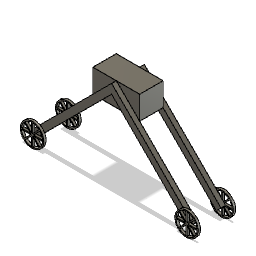
test_5 v1 (Autodesk Fusion 360 design; units mm, degrees)
Autodesk Fusion 360 part; units mm, degrees
sketch "Sketch1" plane through (0, 0, 0) normal (0, 0, 1) x (1, 0, 0)
  line L0 (0, 0) -> (200, 0)
  line L1 (200, 0) -> (200, 100)
  line L2 (200, 100) -> (0, 100)
  line L3 (0, 100) -> (0, 0)
  dimension "d1" = 200
  dimension "d2" = 100
  constraint horizontal L0
  constraint vertical L1
  constraint horizontal L2
  constraint vertical L3
  constraint coincident L0.start L3.end
  measures "d1" distance of L0.start L0.end
  measures "d2" distance of L0.start L2.end
extrude "Extrude1" add sketch "Sketch1" along normal blind 100 makes body 1
move_body "Move1" bodies 1 to x (1, 0, 0) y (0, 1, 0) z (0, 0, 1) at (0, 300, 0)
sketch "Sketch2" plane through (0, 0, 100) normal (0, 0, 1) x (1, 0, 0)
  line L0 (0, 400) -> (0, 300)
  line L1 (0, 300) -> (200, 300)
  line L2 (200, 300) -> (200, 400)
  line L3 (200, 400) -> (0, 400)
  line L4 (100, 400) -> (200, 300)
  line L5 (90, 390) -> (100, 400)
  line L6 (200, 300) -> (190, 290)
  line L7 (100, 400) -> (80, 420)
  line L8 (80, 420) -> (70, 410)
  line L9 (90, 390) -> (0, 300)
  line L10 (100, 400) -> (120, 420)
  line L11 (120, 420) -> (130, 410)
  line L12 (10, 290) -> (0, 300)
  line L13 (190, 290) -> (180, 280)
  line L14 (180, 280) -> (60, 400)
  line L15 (70, 410) -> (60, 400)
  line L16 (130, 410) -> (140, 400)
  line L17 (20, 280) -> (10, 290)
  line L18 (20, 280) -> (140, 400)
  constraint midpoint L3 L4.start
  constraint coincident L1.end L2.start
  constraint perpendicular L4 L5
  constraint perpendicular L5 L7
  constraint perpendicular L7 L8
  constraint coincident L0.end L1.start
  constraint perpendicular L7 L10
  constraint perpendicular L10 L11
  constraint perpendicular L9 L12
  constraint coincident L3 L14.end
  constraint perpendicular L13 L14
  constraint perpendicular L14 L15
  constraint coincident L3 L16.end
  constraint perpendicular L16 L18
extrude "Extrude2" add sketch "Sketch2" along normal blind 20 separate body contours L1 L9 L14 L18 | L1 L12 L17 L18 | L4 L5 L9 L14 L18 | L1 L4 L14 L18 | L1 L6 L13 L14 makes body 2
extrude "Extrude3" add 2 faces at (186.6667, 286.6667, 106.6667) (196.6667, 296.6667, 106.6667) along direction (0.707107, -0.707107, 0) blind 350 separate body on bodies 2 makes body 3
extrude "Extrude4" add 2 faces at (6.6667, 293.3333, 113.3333) (16.6667, 283.3333, 106.6667) along direction (-0.707107, -0.707107, 0) blind 350 separate body on bodies 2 makes body 4
combine "Combine1" operation add target body 4 tool bodies 3 2
sketch "Sketch3" plane through (0, 0, 120) normal (0, 0, 1) x (1, 0, 0)
  line L0 (100, 400) -> (-247.4874, 52.5126)
  line L1 (-247.4874, 52.5126) -> (-227.4874, 32.5126)
  line L2 (-227.4874, 32.5126) -> (100, 360)
  line L3 (100, 360) -> (427.4874, 32.5126)
  line L4 (427.4874, 32.5126) -> (447.4874, 52.5126)
  line L5 (447.4874, 52.5126) -> (100, 400)
  circle A0 centre (-230, 50) radius 50
  circle A1 centre (430, 50) radius 50
  dimension "d11" = 100
  dimension "d12" = 100
  measures "d11" diameter of A0
  measures "d12" diameter of A1
extrude "Extrude5" add sketch "Sketch3" along normal blind 10 separate body contours L0 L1 L2 A0 | L0 L1 L2 A0 | L3 L4 L5 A1 | L3 L4 L5 A1 makes body 5 at (445.235, 35.864, 120) makes body 6 at (-245.0161, 42.7686, 130)
copy_body "CopyPasteBodies1" bodies 4 makes body 7
move_body "Move2" bodies 7 to x (1, 0, 0) y (0, 1, 0) z (0, 0, 1) at (0, 0, -120)
sketch "Sketch4" plane through (0, 0, 130) normal (0, 0, 1) x (1, 0, 0)
  circle A0 centre (-230, 50) radius 50
  line L0 (-230, 100) -> (-230, 0)
  line L1 (-180, 50) -> (-280, 50)
  line L2 (-230, 50) -> (-194.6447, 85.3553)
  line L3 (-230, 50) -> (-180, 50) construction
  line L4 (-230, 50) -> (-194.6447, 14.6447)
  line L5 (-230, 50) -> (-180, 50) construction
  line L6 (-230, 50) -> (-265.3553, 14.6447)
  line L7 (-230, 50) -> (-265.3553, 85.3553)
  circle A1 centre (-230, 50) radius 45
  line L8 (-232.5, 100) -> (-232.5, 0)
  line L9 (-227.5, 100) -> (-227.5, 0)
  line L10 (-231.7678, 51.7678) -> (-196.4124, 87.1231)
  line L11 (-231.7678, 51.7678) -> (-267.1231, 16.4124)
  line L12 (-228.2322, 48.2322) -> (-263.5876, 12.8769)
  line L13 (-228.2322, 48.2322) -> (-192.8769, 83.5876)
  line L14 (-230, 47.5) -> (-180, 47.5)
  arc A2 (-180, 47.5) -> (-180, 52.5) centre (-180, 50) ccw
  line L15 (-180, 52.5) -> (-280, 52.5)
  line L16 (-230, 52.5) -> (-180, 52.5)
  arc A3 (-180, 47.5) -> (-180, 52.5) centre (-180, 50) ccw
  line L17 (-180, 47.5) -> (-280, 47.5)
  line L18 (-228.2322, 51.7678) -> (-263.5876, 87.1231)
  line L19 (-228.2322, 51.7678) -> (-192.8769, 16.4124)
  line L20 (-231.7678, 48.2322) -> (-196.4124, 12.8769)
  line L21 (-231.7678, 48.2322) -> (-267.1231, 83.5876)
  dimension "d15" = 45
  dimension "d16" = 45
  dimension "d17" = 50
  dimension "d18" = -5
  dimension "d19" = 2.5
  dimension "d20" = -2.5
  dimension "d21" = 2.5
  dimension "d22" = -2.5
  dimension "d23" = 2.5
  dimension "d24" = -2.5
  dimension "d25" = 2.5
  dimension "d26" = -2.5
  constraint coincident A0 L0.start
  constraint coincident A0 L0.end
  constraint vertical L0
  constraint coincident A0 L1.start
  constraint coincident A0 L1.end
  constraint perpendicular L0 L1
  constraint horizontal L3
  constraint coincident A0.centre L2.start
  constraint horizontal L5
  constraint coincident A0 L6.end
  constraint perpendicular L4 L6
  constraint coincident A0 L7.end
  constraint perpendicular L6 L7
  measures "d15" angle of L2 L3
  measures "d16" angle of L4 L5
  measures "d17" distance of A0.centre L4.end
extrude "Extrude6" cut sketch "Sketch4" against normal blind 10 contours A1 L13 L15 L16 | A1 L14 L17 L19 | A1 L9 L10 | A1 L9 L20 | A1 L8 L18 | A1 L8 L12 | A1 L11 L17 | A1 L15 L21 bodies 6
delete_body "RemoveBody1" bodies 5
copy_body "CopyPasteBodies3" bodies 6 makes body 8
copy_body "CopyPasteBodies4" bodies 6 makes body 9
move_body "Move4" bodies 9 to x (1, 0, 0) y (0, 1, 0) z (0, 0, 1) at (0, 0, -150)
copy_body "CopyPasteBodies5" bodies 8 9 makes body 10 makes body 11
move_body "Move5" bodies 10 11 to x (1, 0, 0) y (0, 1, 0) z (0, 0, 1) at (660, 0, 0)
